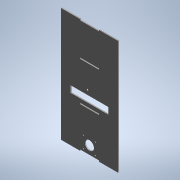
# Autodesk Inventor part: MuurR
Saved by Autodesk Inventor 2020 (Build 240168000, 168)
## iProperties
Part Number: MuurR
Material: Generic
Document SubType Name: Modeling
Designer: SBBA
Appearance: Default
Mass: 126.51 g
Surface Area: 890.564 cm^2
Volume: 126.51 cm^3
Density: 1 g/cm^3
Author: SBBA
Autodesk Inventor part; units mm, degrees
ref_plane "YZ Plane" through (0, 0, 0) normal (1, 0, 0) x (0, 1, 0)
ref_plane "XZ Plane" through (0, 0, 0) normal (0, 1, 0) x (-1, 0, 0)
ref_plane "XY Plane" through (0, 0, 0) normal (0, 0, 1) x (1, 0, 0)
sketch "Sketch1" plane through (0, 0, 0) normal (0, 0, 1) x (1, 0, 0)
  line L0 (-70.3712, 150.7033) -> (79.6288, 150.7033)
  line L1 (79.6288, 150.7033) -> (79.6288, -149.2967)
  line L2 (79.6288, -149.2967) -> (-70.3712, -149.2967)
  line L3 (-70.3712, -149.2967) -> (-70.3712, 150.7033)
  point P0 (0, 0)
  constraints: 8 end point, 2 parallel, 1 horizontal, 1 perpendicular
extrude "Extrusion1" add sketch "Sketch1" along normal blind 3
sketch "Sketch2" plane through (0, 0, 3) normal (0, 0, 1) x (1, 0, 0)
  line L0 (-70.3712, 150.7033) -> (-70.3712, -149.2967) projected
  line L1 (-70.3712, 271.0495) -> (-120.3712, 271.0495)
  line L2 (-20.3712, 147.7184) -> (-20.3712, 150.7184)
  line L3 (-20.3712, 147.7184) -> (29.6288, 147.7184)
  line L4 (29.6288, 147.7184) -> (29.6288, 150.7184)
  line L5 (-20.3712, 150.7184) -> (29.6288, 150.7184)
  line L6 (79.6288, 150.7033) -> (-70.3712, 150.7033) projected
  point P0 (0, 0)
  dimension "d9" = 50
  constraints: 10 end point, 2 horizontal, 2 vertical, 1 parallel, 1 point on line
  measures "d9" distance of L1.start L1.end
extrude "Extrusion2" cut sketch "Sketch2" against normal blind 3
sketch "Sketch3" plane through (0, 0, 3) normal (0, 0, 1) x (1, 0, 0)
  line L0 (-20.3712, 150.7033) -> (-20.3712, 147.7184) projected
  line L1 (-20.3712, -149.2722) -> (29.6288, -149.2967)
  line L2 (79.6288, -149.2967) -> (-70.3712, -149.2967) projected
  line L3 (-20.3712, -149.2722) -> (-20.3712, -146.2722)
  line L4 (-20.3712, -146.2722) -> (29.6288, -146.2967)
  line L5 (29.6288, -146.2967) -> (29.6288, -149.2967)
  point P0 (0, 0)
  constraints: 8 end point, 1 point on line, 1 vertical
extrude "Extrusion3" cut sketch "Sketch3" against normal blind 3
sketch "Sketch4" plane through (0, 0, 3) normal (0, 0, 1) x (1, 0, 0)
  line L0 (29.6288, -46.2722) -> (-20.3712, -46.2722)
  line L1 (-20.3712, -46.2722) -> (29.6288, -46.2722)
  line L2 (29.6288, -46.2722) -> (29.6288, -43.6172)
  line L3 (29.6288, -43.6172) -> (-20.3712, -43.6172)
  line L4 (-20.3712, -43.6172) -> (-20.3712, -46.2722)
  point P0 (0, 0)
  constraints: 10 end point, 2 parallel, 1 horizontal, 1 perpendicular
extrude "Extrusion4" add sketch "Sketch4" against normal blind 3
sketch "Sketch5" plane through (0, 0, 3) normal (0, 0, 1) x (1, 0, 0)
  line L0 (-20.3712, -42.9205) -> (29.6288, -42.9205)
  line L1 (29.6288, -42.9205) -> (29.6288, -39.9205)
  line L2 (29.6288, -39.9205) -> (-20.3712, -39.9205)
  line L3 (-20.3712, -39.9205) -> (-20.3712, -42.9205)
  point P0 (0, 0)
  point P1 (-20.3712, -146.2722)
  point P2 (29.6288, -146.2967)
  constraints: 8 end point, 2 parallel, 1 horizontal, 1 perpendicular
extrude "Extrusion5" cut sketch "Sketch5" against normal blind 3
sketch "Sketch6" plane through (0, 0, 3) normal (0, 0, 1) x (1, 0, 0)
  line L0 (29.6288, -39.9205) -> (-20.3712, -39.9205) projected
  line L1 (-20.3712, 60.1524) -> (29.6288, 60.1524)
  line L2 (29.6288, 60.1524) -> (29.6288, 63.1524)
  line L3 (29.6288, 63.1524) -> (-20.3712, 63.1524)
  line L4 (-20.3712, 63.1524) -> (-20.3712, 60.1524)
  point P0 (0, 0)
  constraints: 8 end point, 2 parallel, 1 horizontal, 1 perpendicular
extrude "Extrusion6" cut sketch "Sketch6" against normal blind 3
sketch "Sketch7" plane through (0, 0, 3) normal (0, 0, 1) x (1, 0, 0)
  line L0 (29.6288, -149.2967) -> (-70.3712, -149.2967) projected
  line L1 (-70.3712, -149.2967) -> (-70.3712, 150.7033) projected
  circle A0 centre (4.6288, -99.2967) radius 12
  point P0 (0, 0)
  constraints: 1 centre point
extrude "Extrusion7" cut sketch "Sketch7" against normal blind 3
sketch "Sketch8" plane through (0, 0, 3) normal (0, 0, 1) x (1, 0, 0)
  circle A0 centre (4.6288, -99.2967) radius 12 projected
  circle A1 centre (20.6853, -83.2968) radius 1.5
  circle A2 centre (-11.3147, -83.2968) radius 1.5
  circle A3 centre (-11.3712, -115.2967) radius 1.5
  circle A4 centre (20.6288, -115.2967) radius 1.5
  point P0 (0, 0)
  constraints: 4 centre point
extrude "Extrusion8" cut sketch "Sketch8" against normal blind 3 contours A1 | A2 | A3 | A4
sketch "Sketch9" plane through (0, 0, 3) normal (0, 0, 1) x (1, 0, 0)
  point P0 (0, 0)
sketch "Sketch11" plane through (0, 0, 3) normal (0, 0, 1) x (1, 0, 0)
  line L0 (-20.3712, -39.9205) -> (29.6288, -39.9205) projected
  line L1 (79.6288, -149.2967) -> (79.6288, 150.7033) projected
  line L2 (-70.3712, 150.7033) -> (-70.3712, -149.2967) projected
  line L3 (29.6288, 60.1524) -> (-20.3712, 60.1524) projected
  line L4 (-45.3712, -29.9205) -> (54.6288, -29.9205)
  line L5 (54.6288, -29.9205) -> (54.6288, -12.4205)
  line L6 (54.6288, -12.4205) -> (-45.3712, -12.4205)
  line L7 (-45.3712, -12.4205) -> (-45.3712, -29.9205)
  point P0 (0, 0)
  constraints: 8 end point, 2 parallel, 1 horizontal, 1 perpendicular
extrude "Extrusion9" cut sketch "Sketch11" against normal blind 10.5
sketch "Sketch12" plane through (0, 0, 3) normal (0, 0, 1) x (1, 0, 0)
  circle A0 centre (4.6288, -99.2967) radius 12 projected
  circle A1 centre (4.6288, -99.2967) radius 29.508
  point P0 (0, 0)
  constraints: 1 centre point, 1 coincident
extrude "Extrusion10" cut sketch "Sketch12" against normal blind 11.75
sketch "Sketch13" plane through (0, 0, 3) normal (0, 0, 1) x (1, 0, 0)
  circle A0 centre (4.6288, -99.2967) radius 29.508 projected
  circle A1 centre (4.6288, -99.2967) radius 29.508
  point P0 (0, 0)
  constraints: 1 centre point, 1 coincident
extrude "Extrusion11" add sketch "Sketch13" against normal blind 3
sketch "Sketch14" plane through (29.6288, -149.2967, 3) normal (0.0005, 1, 0) x (1, -0.0005, 0)
  line L0 (-100, 0) -> (0, 0) projected
  line L1 (-0.0015, 3) -> (-50.0015, 3) projected
  line L2 (-50, 0) -> (-0.0015, 0)
  line L3 (-0.0015, 0) -> (-0.0015, 3)
  line L4 (-0.0015, 3) -> (-50, 3)
  line L5 (-50, 3) -> (-50, 0)
  point P0 (-29.7019, 3)
  constraints: 8 end point, 2 parallel, 1 horizontal, 1 midpoint, 1 perpendicular
extrude "Extrusion12" cut sketch "Sketch14" against normal blind 16.25
sketch "Sketch15" plane through (0, 0, 3) normal (0, 0, 1) x (1, 0, 0)
  line L0 (-20.3712, -146.2722) -> (29.6288, -146.2967) projected
  circle A0 centre (-10.8712, -109.2844) radius 1.5
  circle A1 centre (20.1288, -109.2844) radius 1.5
  circle A2 centre (20.1288, -140.2844) radius 1.5
  circle A3 centre (-10.8712, -140.2844) radius 1.5
  circle A4 centre (4.6288, -124.7844) radius 12
  point P0 (0, 0)
  constraints: 5 centre point
extrude "Extrusion13" cut sketch "Sketch15" against normal blind 21.5
body "Solid1"
